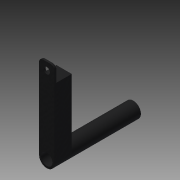
# Autodesk Inventor part: Rod Spacer
Saved by Autodesk Inventor 2015 (Build 190159000, 159)
## iProperties
Created: 2015-10-19
Part Number: Rod Spacer
Material: ABS Plastic
Document SubType Name: Modeling
Designer: James
Density: 1.06 g/cm^3
Appearance: Smooth - White
Author: James
Autodesk Inventor part; units mm, degrees
ref_plane "YZ Plane" through (0, 0, 0) normal (1, 0, 0) x (0, 1, 0)
ref_plane "XZ Plane" through (0, 0, 0) normal (0, 1, 0) x (-1, 0, 0)
ref_plane "XY Plane" through (0, 0, 0) normal (0, 0, 1) x (1, 0, 0)
sketch "Sketch1" plane through (0, 0, 0) normal (0, 1, 0) x (-1, 0, 0)
  circle A0 centre (0, 0) radius 3
  circle A1 centre (0, 0) radius 4
  dimension "d0" = 6
  dimension "d1" = 8
  constraints: 2 centre point, 2 coincident
  measures "d0" diameter of A0
  measures "d1" diameter of A1
extrude "Extrusion1" add sketch "Sketch1" along normal blind 45
sketch "Sketch2" plane through (0, 0, 0) normal (0, 1, 0) x (-1, 0, 0)
  circle A0 centre (0, 0) radius 4 projected
  line L0 (-4, 0) -> (-4, 42)
  line L1 (-2, 44) -> (2, 44)
  line L2 (4, 42) -> (4, 0)
  arc A1 (-2, 44) -> (-4, 42) centre (-2, 42) ccw
  arc A2 (4, 42) -> (2, 44) centre (2, 42) ccw
  circle A3 centre (0, 40) radius 1.65
  point P0 (-4, 44)
  point P1 (4, 44)
  dimension "d4" = 44
  dimension "d5" = 8
  dimension "d6" = 2
  dimension "d10" = 3.3
  constraints: 6 end point, 6 point on circle, 6 tangent, 4 point on line, 3 centre point, 1 equal radius, 1 perpendicular, 1 vertical
  measures "d4" distance of L0.start point (-4, 44)
  measures "d5" distance of point (-4, 44) point (4, 44)
  measures "d6" radius of A1
  measures "d10" diameter of A3
extrude "Extrusion2" add sketch "Sketch2" along normal blind 10 contours A0 L0 A1 L1 A2 L2
chamfer "Chamfer1" distance 1 angle 45 5 edges at (4, 10, 21) (3.4142, 10, 43.4142) (0, 10, 44) (-3.4142, 10, 43.4142) (-4, 10, 21)
sketch "Sketch4" plane through (0, 10, 0) normal (0, 1, 0) x (1, 0, 0)
  circle A0 centre (0, -40) radius 1.65 projected
  line L0 (4, -36) -> (-4, -36)
  line L1 (-4, -36) -> (-4, -44)
  line L2 (-4, -44) -> (4, -44)
  line L3 (4, -44) -> (4, -36)
  line L4 (4, -36) -> (-4, -44) construction
  line L5 (-4, -36) -> (4, -44) construction
  point P0 (0, 0)
  point P1 (-2, -44)
  point P2 (-4, -42)
  constraints: 12 end point, 2 midpoint, 2 parallel, 1 horizontal, 1 perpendicular
extrude "Extrusion3" cut sketch "Sketch4" against normal blind 9
chamfer "Chamfer4" distance 1 angle 45 1 edges at (0, 10, 36)
body "Solid1"
